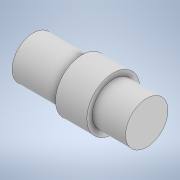
# Autodesk Inventor part: Валл_резина
Saved by Autodesk Inventor 2021 (Build 250183000, 183)
## iProperties
Created: 2023-04-28
Part Number: Валл_резина
Material: Типовые
Document SubType Name: Modeling
Designer: gdevc
Density: 1 g/cm^3
Appearance: По умолчанию
Mass: 19.4411 g
Surface Area: 45.7926 cm^2
Volume: 19.4411 cm^3
Author: gdevc
Autodesk Inventor part; units mm, degrees
ref_plane "YZ Plane" through (0, 0, 0) normal (1, 0, 0) x (0, 1, 0)
ref_plane "XZ Plane" through (0, 0, 0) normal (0, 1, 0) x (-1, 0, 0)
ref_plane "XY Plane" through (0, 0, 0) normal (0, 0, 1) x (1, 0, 0)
sketch "Эскиз1" plane through (0, 0, 0) normal (0, 0, 1) x (1, 0, 0)
  line L0 (0, 0) -> (53.555, 0)
  line L1 (0, 0) -> (0, 10)
  line L2 (37.805, 12.5) -> (37.805, 10)
  line L3 (37.805, 10) -> (53.555, 10)
  line L4 (53.555, 10) -> (53.555, 0)
  line L5 (2, 10) -> (2, 10)
  line L6 (2, 10) -> (23, 10)
  line L7 (23, 10) -> (23, 12.5)
  line L8 (0, 10) -> (2, 10)
  line L9 (23, 12.5) -> (37.805, 12.5)
  dimension "d0" = 20
  dimension "d2" = 15.75
  dimension "d5" = 20
  dimension "d6" = 21
  dimension "d7" = 2
  dimension "d8" = 20
  dimension "d9" = 25
  dimension "d10" = 37.805
  constraints: 20 end point, 9 perpendicular, 2 vertical, 1 horizontal
  measures "d0" diameter of L3 L0
  measures "d2" distance of L2.end L3.end
  measures "d5" diameter of L6 L0
  measures "d6" distance between parallel lines of L7 L5
  measures "d7" distance between parallel lines of L1 L5
  measures "d8" diameter of L8 L0
  measures "d9" diameter of L9 L0
  measures "d10" distance from line of L0.start L2
revolve "Вращение1" add sketch "Эскиз1" angle 360 about axis through (0, 0, 0) along (1, 0, 0)
